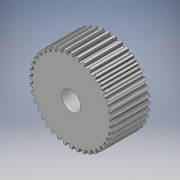
# Autodesk Inventor part: engranaje_grande_1
Saved by Autodesk Inventor 2017 (Build 210142000, 142)
## iProperties
Created: 2016-10-04
Part Number: engranaje_grande_1
Material: Generic
Document SubType Name: Modeling
Designer: ANDRES
Density: 1 g/cm^3
Appearance: Default
Author: ANDRES
Autodesk Inventor part; units mm, degrees
(part 1 of 2)
ref_plane "YZ Plane" through (0, 0, 0) normal (1, 0, 0) x (0, 1, 0)
ref_plane "XZ Plane" through (0, 0, 0) normal (0, 1, 0) x (-1, 0, 0)
ref_plane "XY Plane" through (0, 0, 0) normal (0, 0, 1) x (1, 0, 0)
sketch "Sketch1" plane through (0, 0, 0) normal (0, 1, 0) x (-1, 0, 0)
  line L0 (2.1221, 1.1536) -> (2.1255, 1.153)
  line L1 (2.1255, 1.153) -> (2.1288, 1.1523)
  line L2 (2.1288, 1.1523) -> (2.1356, 1.1509)
  line L3 (2.1356, 1.1509) -> (2.1491, 1.1475)
  line L4 (2.1491, 1.1475) -> (2.1626, 1.1435)
  line L5 (2.1626, 1.1435) -> (2.1761, 1.1388)
  line L6 (2.1761, 1.1388) -> (2.1896, 1.1337)
  line L7 (2.1896, 1.1337) -> (2.2031, 1.128)
  line L8 (2.2031, 1.128) -> (2.2031, 1.0754)
  line L9 (2.2031, 1.0754) -> (2.1896, 1.0697)
  line L10 (2.1896, 1.0697) -> (2.1761, 1.0646)
  line L11 (2.1761, 1.0646) -> (2.1626, 1.06)
  line L12 (2.1626, 1.06) -> (2.1491, 1.0559)
  line L13 (2.1491, 1.0559) -> (2.1356, 1.0525)
  line L14 (2.1356, 1.0525) -> (2.1288, 1.0511)
  line L15 (2.1288, 1.0511) -> (2.1255, 1.0505)
  line L16 (2.1255, 1.0505) -> (2.1221, 1.0499)
  line L17 (2.1221, 1.0499) -> (2.1176, 0.9933)
  line L18 (2.1176, 0.9933) -> (2.1209, 0.9922)
  line L19 (2.1209, 0.9922) -> (2.1241, 0.991)
  line L20 (2.1241, 0.991) -> (2.1305, 0.9885)
  line L21 (2.1305, 0.9885) -> (2.1433, 0.9831)
  line L22 (2.1433, 0.9831) -> (2.1561, 0.977)
  line L23 (2.1561, 0.977) -> (2.1687, 0.9703)
  line L24 (2.1687, 0.9703) -> (2.1812, 0.9631)
  line L25 (2.1812, 0.9631) -> (2.1936, 0.9554)
  line L26 (2.1936, 0.9554) -> (2.1854, 0.9034)
  line L27 (2.1854, 0.9034) -> (2.1712, 0.8999)
  line L28 (2.1712, 0.8999) -> (2.1571, 0.897)
  line L29 (2.1571, 0.897) -> (2.143, 0.8945)
  line L30 (2.143, 0.8945) -> (2.129, 0.8926)
  line L31 (2.129, 0.8926) -> (2.1151, 0.8914)
  line L32 (2.1151, 0.8914) -> (2.1083, 0.891)
  line L33 (2.1083, 0.891) -> (2.1048, 0.8909)
  line L34 (2.1048, 0.8909) -> (2.1014, 0.8909)
  line L35 (2.1014, 0.8909) -> (2.0882, 0.8357)
  line L36 (2.0882, 0.8357) -> (2.0912, 0.8341)
  line L37 (2.0912, 0.8341) -> (2.0942, 0.8324)
  line L38 (2.0942, 0.8324) -> (2.1002, 0.829)
  line L39 (2.1002, 0.829) -> (2.112, 0.8216)
  line L40 (2.112, 0.8216) -> (2.1236, 0.8136)
  line L41 (2.1236, 0.8136) -> (2.135, 0.805)
  line L42 (2.135, 0.805) -> (2.1462, 0.7959)
  line L43 (2.1462, 0.7959) -> (2.1573, 0.7864)
  line L44 (2.1573, 0.7864) -> (2.1411, 0.7363)
  line L45 (2.1411, 0.7363) -> (2.1265, 0.7351)
  line L46 (2.1265, 0.7351) -> (2.112, 0.7344)
  line L47 (2.112, 0.7344) -> (2.0978, 0.7342)
  line L48 (2.0978, 0.7342) -> (2.0837, 0.7345)
  line L49 (2.0837, 0.7345) -> (2.0698, 0.7355)
  line L50 (2.0698, 0.7355) -> (2.0629, 0.7362)
  line L51 (2.0629, 0.7362) -> (2.0595, 0.7366)
  line L52 (2.0595, 0.7366) -> (2.0561, 0.7371)
  line L53 (2.0561, 0.7371) -> (2.0344, 0.6847)
  line L54 (2.0344, 0.6847) -> (2.0371, 0.6826)
  line L55 (2.0371, 0.6826) -> (2.0398, 0.6805)
  line L56 (2.0398, 0.6805) -> (2.0452, 0.6762)
  line L57 (2.0452, 0.6762) -> (2.0557, 0.667)
  line L58 (2.0557, 0.667) -> (2.0659, 0.6573)
  line L59 (2.0659, 0.6573) -> (2.0759, 0.647)
  line L60 (2.0759, 0.647) -> (2.0856, 0.6363)
  line L61 (2.0856, 0.6363) -> (2.095, 0.6251)
  line L62 (2.095, 0.6251) -> (2.0711, 0.5783)
  line L63 (2.0711, 0.5783) -> (2.0565, 0.5793)
  line L64 (2.0565, 0.5793) -> (2.0421, 0.5808)
  line L65 (2.0421, 0.5808) -> (2.028, 0.5829)
  line L66 (2.028, 0.5829) -> (2.0141, 0.5854)
  line L67 (2.0141, 0.5854) -> (2.0006, 0.5885)
  line L68 (2.0006, 0.5885) -> (1.9939, 0.5903)
  line L69 (1.9939, 0.5903) -> (1.9906, 0.5913)
  line L70 (1.9906, 0.5913) -> (1.9873, 0.5923)
  line L71 (1.9873, 0.5923) -> (1.9577, 0.5439)
  line L72 (1.9577, 0.5439) -> (1.9601, 0.5414)
  line L73 (1.9601, 0.5414) -> (1.9624, 0.5389)
  line L74 (1.9624, 0.5389) -> (1.967, 0.5338)
  line L75 (1.967, 0.5338) -> (1.976, 0.5231)
  line L76 (1.976, 0.5231) -> (1.9845, 0.5119)
  line L77 (1.9845, 0.5119) -> (1.9927, 0.5002)
  line L78 (1.9927, 0.5002) -> (2.0006, 0.4881)
  line L79 (2.0006, 0.4881) -> (2.0082, 0.4756)
  line L80 (2.0082, 0.4756) -> (1.9773, 0.4331)
  line L81 (1.9773, 0.4331) -> (1.963, 0.4364)
  line L82 (1.963, 0.4364) -> (1.9491, 0.4401)
  line L83 (1.9491, 0.4401) -> (1.9354, 0.4444)
  line L84 (1.9354, 0.4444) -> (1.9221, 0.449)
  line L85 (1.9221, 0.449) -> (1.9092, 0.4542)
  line L86 (1.9092, 0.4542) -> (1.9029, 0.457)
  line L87 (1.9029, 0.457) -> (1.8998, 0.4585)
  line L88 (1.8998, 0.4585) -> (1.8967, 0.46)
  line L89 (1.8967, 0.46) -> (1.8599, 0.4168)
  line L90 (1.8599, 0.4168) -> (1.8619, 0.414)
  line L91 (1.8619, 0.414) -> (1.8638, 0.4112)
  line L92 (1.8638, 0.4112) -> (1.8675, 0.4054)
  line L93 (1.8675, 0.4054) -> (1.8747, 0.3935)
  line L94 (1.8747, 0.3935) -> (1.8814, 0.3811)
  line L95 (1.8814, 0.3811) -> (1.8877, 0.3683)
  line L96 (1.8877, 0.3683) -> (1.8936, 0.3551)
  line L97 (1.8936, 0.3551) -> (1.8991, 0.3415)
  line L98 (1.8991, 0.3415) -> (1.8619, 0.3043)
  line L99 (1.8619, 0.3043) -> (1.8484, 0.3098)
  line L100 (1.8484, 0.3098) -> (1.8352, 0.3157)
  line L101 (1.8352, 0.3157) -> (1.8223, 0.322)
  line L102 (1.8223, 0.322) -> (1.8099, 0.3287)
  line L103 (1.8099, 0.3287) -> (1.798, 0.3359)
  line L104 (1.798, 0.3359) -> (1.7922, 0.3396)
  line L105 (1.7922, 0.3396) -> (1.7894, 0.3416)
  line L106 (1.7894, 0.3416) -> (1.7866, 0.3435)
  line L107 (1.7866, 0.3435) -> (1.7434, 0.3067)
  line L108 (1.7434, 0.3067) -> (1.7449, 0.3036)
  line L109 (1.7449, 0.3036) -> (1.7464, 0.3005)
  line L110 (1.7464, 0.3005) -> (1.7492, 0.2942)
  line L111 (1.7492, 0.2942) -> (1.7544, 0.2813)
  line L112 (1.7544, 0.2813) -> (1.7591, 0.268)
  line L113 (1.7591, 0.268) -> (1.7633, 0.2543)
  line L114 (1.7633, 0.2543) -> (1.767, 0.2404)
  line L115 (1.767, 0.2404) -> (1.7704, 0.2261)
  line L116 (1.7704, 0.2261) -> (1.7278, 0.1952)
  line L117 (1.7278, 0.1952) -> (1.7153, 0.2028)
  line L118 (1.7153, 0.2028) -> (1.7032, 0.2107)
  line L119 (1.7032, 0.2107) -> (1.6915, 0.2189)
  line L120 (1.6915, 0.2189) -> (1.6803, 0.2275)
  line L121 (1.6803, 0.2275) -> (1.6696, 0.2364)
  line L122 (1.6696, 0.2364) -> (1.6645, 0.241)
  line L123 (1.6645, 0.241) -> (1.662, 0.2434)
  line L124 (1.662, 0.2434) -> (1.6595, 0.2457)
  line L125 (1.6595, 0.2457) -> (1.6112, 0.2161)
  line L126 (1.6112, 0.2161) -> (1.6121, 0.2128)
  line L127 (1.6121, 0.2128) -> (1.6131, 0.2095)
  line L128 (1.6131, 0.2095) -> (1.6149, 0.2029)
  line L129 (1.6149, 0.2029) -> (1.618, 0.1893)
  line L130 (1.618, 0.1893) -> (1.6205, 0.1754)
  line L131 (1.6205, 0.1754) -> (1.6226, 0.1613)
  line L132 (1.6226, 0.1613) -> (1.6241, 0.1469)
  line L133 (1.6241, 0.1469) -> (1.6252, 0.1323)
  line L134 (1.6252, 0.1323) -> (1.5783, 0.1084)
  line L135 (1.5783, 0.1084) -> (1.5671, 0.1179)
  line L136 (1.5671, 0.1179) -> (1.5564, 0.1275)
  line L137 (1.5564, 0.1275) -> (1.5461, 0.1375)
  line L138 (1.5461, 0.1375) -> (1.5364, 0.1477)
  line L139 (1.5364, 0.1477) -> (1.5273, 0.1582)
  line L140 (1.5273, 0.1582) -> (1.5229, 0.1636)
  line L141 (1.5229, 0.1636) -> (1.5208, 0.1663)
  line L142 (1.5208, 0.1663) -> (1.5188, 0.169)
  line L143 (1.5188, 0.169) -> (1.4663, 0.1473)
  line L144 (1.4663, 0.1473) -> (1.4668, 0.1439)
  line L145 (1.4668, 0.1439) -> (1.4672, 0.1405)
  line L146 (1.4672, 0.1405) -> (1.468, 0.1336)
  line L147 (1.468, 0.1336) -> (1.4689, 0.1197)
  line L148 (1.4689, 0.1197) -> (1.4692, 0.1056)
  line L149 (1.4692, 0.1056) -> (1.469, 0.0914)
  line L150 (1.469, 0.0914) -> (1.4683, 0.0769)
  line L151 (1.4683, 0.0769) -> (1.4671, 0.0624)
  line L152 (1.4671, 0.0624) -> (1.417, 0.0461)
  line L153 (1.417, 0.0461) -> (1.4075, 0.0572)
  line L154 (1.4075, 0.0572) -> (1.3984, 0.0684)
  line L155 (1.3984, 0.0684) -> (1.3898, 0.0799)
  line L156 (1.3898, 0.0799) -> (1.3818, 0.0915)
  line L157 (1.3818, 0.0915) -> (1.3744, 0.1033)
  line L158 (1.3744, 0.1033) -> (1.371, 0.1092)
  line L159 (1.371, 0.1092) -> (1.3693, 0.1122)
  line L160 (1.3693, 0.1122) -> (1.3677, 0.1153)
  line L161 (1.3677, 0.1153) -> (1.3125, 0.102)
  line L162 (1.3125, 0.102) -> (1.3125, 0.0986)
  line L163 (1.3125, 0.0986) -> (1.3124, 0.0952)
  line L164 (1.3124, 0.0952) -> (1.312, 0.0883)
  line L165 (1.312, 0.0883) -> (1.3108, 0.0744)
  line L166 (1.3108, 0.0744) -> (1.3089, 0.0604)
  line L167 (1.3089, 0.0604) -> (1.3065, 0.0464)
  line L168 (1.3065, 0.0464) -> (1.3035, 0.0322)
  line L169 (1.3035, 0.0322) -> (1.3, 0.018)
  line L170 (1.3, 0.018) -> (1.248, 0.0098)
  line L171 (1.248, 0.0098) -> (1.2403, 0.0222)
  line L172 (1.2403, 0.0222) -> (1.2331, 0.0347)
  line L173 (1.2331, 0.0347) -> (1.2264, 0.0474)
  line L174 (1.2264, 0.0474) -> (1.2203, 0.0601)
  line L175 (1.2203, 0.0601) -> (1.2149, 0.0729)
  line L176 (1.2149, 0.0729) -> (1.2124, 0.0793)
  line L177 (1.2124, 0.0793) -> (1.2112, 0.0825)
  line L178 (1.2112, 0.0825) -> (1.2101, 0.0858)
  line L179 (1.2101, 0.0858) -> (1.1536, 0.0813)
  line L180 (1.1536, 0.0813) -> (1.153, 0.078)
  line L181 (1.153, 0.078) -> (1.1523, 0.0746)
  line L182 (1.1523, 0.0746) -> (1.1509, 0.0678)
  line L183 (1.1509, 0.0678) -> (1.1475, 0.0543)
  line L184 (1.1475, 0.0543) -> (1.1435, 0.0408)
  line L185 (1.1435, 0.0408) -> (1.1388, 0.0273)
  line L186 (1.1388, 0.0273) -> (1.1337, 0.0138)
  line L187 (1.1337, 0.0138) -> (1.128, 0.0003)
  line L188 (1.128, 0.0003) -> (1.0754, 0.0003)
  line L189 (1.0754, 0.0003) -> (1.0697, 0.0138)
  line L190 (1.0697, 0.0138) -> (1.0646, 0.0273)
  line L191 (1.0646, 0.0273) -> (1.06, 0.0408)
  line L192 (1.06, 0.0408) -> (1.0559, 0.0543)
  line L193 (1.0559, 0.0543) -> (1.0525, 0.0678)
  line L194 (1.0525, 0.0678) -> (1.0511, 0.0746)
  line L195 (1.0511, 0.0746) -> (1.0505, 0.078)
  line L196 (1.0505, 0.078) -> (1.0499, 0.0813)
  line L197 (1.0499, 0.0813) -> (0.9933, 0.0858)
  line L198 (0.9933, 0.0858) -> (0.9922, 0.0825)
  line L199 (0.9922, 0.0825) -> (0.991, 0.0793)
  line L200 (0.991, 0.0793) -> (0.9885, 0.0729)
  line L201 (0.9885, 0.0729) -> (0.9831, 0.0601)
  line L202 (0.9831, 0.0601) -> (0.977, 0.0474)
  line L203 (0.977, 0.0474) -> (0.9703, 0.0347)
  line L204 (0.9703, 0.0347) -> (0.9631, 0.0222)
  line L205 (0.9631, 0.0222) -> (0.9554, 0.0098)
  line L206 (0.9554, 0.0098) -> (0.9034, 0.018)
  line L207 (0.9034, 0.018) -> (0.8999, 0.0322)
  line L208 (0.8999, 0.0322) -> (0.897, 0.0464)
  line L209 (0.897, 0.0464) -> (0.8945, 0.0604)
  line L210 (0.8945, 0.0604) -> (0.8926, 0.0744)
  line L211 (0.8926, 0.0744) -> (0.8914, 0.0883)
  line L212 (0.8914, 0.0883) -> (0.891, 0.0952)
  line L213 (0.891, 0.0952) -> (0.8909, 0.0986)
  line L214 (0.8909, 0.0986) -> (0.8909, 0.102)
  line L215 (0.8909, 0.102) -> (0.8357, 0.1153)
  line L216 (0.8357, 0.1153) -> (0.8341, 0.1122)
  line L217 (0.8341, 0.1122) -> (0.8324, 0.1092)
  line L218 (0.8324, 0.1092) -> (0.829, 0.1033)
  line L219 (0.829, 0.1033) -> (0.8216, 0.0915)
  line L220 (0.8216, 0.0915) -> (0.8136, 0.0799)
  line L221 (0.8136, 0.0799) -> (0.805, 0.0684)
  line L222 (0.805, 0.0684) -> (0.7959, 0.0572)
  line L223 (0.7959, 0.0572) -> (0.7864, 0.0461)
  line L224 (0.7864, 0.0461) -> (0.7363, 0.0624)
  line L225 (0.7363, 0.0624) -> (0.7351, 0.0769)
  line L226 (0.7351, 0.0769) -> (0.7344, 0.0914)
  line L227 (0.7344, 0.0914) -> (0.7342, 0.1056)
  line L228 (0.7342, 0.1056) -> (0.7345, 0.1197)
  line L229 (0.7345, 0.1197) -> (0.7355, 0.1336)
  line L230 (0.7355, 0.1336) -> (0.7362, 0.1405)
  line L231 (0.7362, 0.1405) -> (0.7366, 0.1439)
  line L232 (0.7366, 0.1439) -> (0.7371, 0.1473)
  line L233 (0.7371, 0.1473) -> (0.6847, 0.169)
  line L234 (0.6847, 0.169) -> (0.6826, 0.1663)
  line L235 (0.6826, 0.1663) -> (0.6805, 0.1636)
  line L236 (0.6805, 0.1636) -> (0.6762, 0.1582)
  line L237 (0.6762, 0.1582) -> (0.667, 0.1477)
  line L238 (0.667, 0.1477) -> (0.6573, 0.1375)
  line L239 (0.6573, 0.1375) -> (0.647, 0.1275)
  line L240 (0.647, 0.1275) -> (0.6363, 0.1179)
  line L241 (0.6363, 0.1179) -> (0.6251, 0.1084)
  line L242 (0.6251, 0.1084) -> (0.5783, 0.1323)
  line L243 (0.5783, 0.1323) -> (0.5793, 0.1469)
  line L244 (0.5793, 0.1469) -> (0.5808, 0.1613)
  line L245 (0.5808, 0.1613) -> (0.5829, 0.1754)
  line L246 (0.5829, 0.1754) -> (0.5854, 0.1893)
  line L247 (0.5854, 0.1893) -> (0.5885, 0.2029)
  line L248 (0.5885, 0.2029) -> (0.5903, 0.2095)
  line L249 (0.5903, 0.2095) -> (0.5913, 0.2128)
  line L250 (0.5913, 0.2128) -> (0.5923, 0.2161)
  line L251 (0.5923, 0.2161) -> (0.5439, 0.2457)
  line L252 (0.5439, 0.2457) -> (0.5414, 0.2434)
  line L253 (0.5414, 0.2434) -> (0.5389, 0.241)
  line L254 (0.5389, 0.241) -> (0.5338, 0.2364)
  line L255 (0.5338, 0.2364) -> (0.5231, 0.2275)
  line L256 (0.5231, 0.2275) -> (0.5119, 0.2189)
  line L257 (0.5119, 0.2189) -> (0.5002, 0.2107)
  line L258 (0.5002, 0.2107) -> (0.4881, 0.2028)
  line L259 (0.4881, 0.2028) -> (0.4756, 0.1952)
  line L260 (0.4756, 0.1952) -> (0.4331, 0.2261)
  line L261 (0.4331, 0.2261) -> (0.4364, 0.2404)
  line L262 (0.4364, 0.2404) -> (0.4401, 0.2543)
  line L263 (0.4401, 0.2543) -> (0.4444, 0.268)
  line L264 (0.4444, 0.268) -> (0.449, 0.2813)
  line L265 (0.449, 0.2813) -> (0.4542, 0.2942)
  line L266 (0.4542, 0.2942) -> (0.457, 0.3005)
  line L267 (0.457, 0.3005) -> (0.4585, 0.3036)
  line L268 (0.4585, 0.3036) -> (0.46, 0.3067)
  line L269 (0.46, 0.3067) -> (0.4168, 0.3435)
  line L270 (0.4168, 0.3435) -> (0.414, 0.3416)
  line L271 (0.414, 0.3416) -> (0.4112, 0.3396)
  line L272 (0.4112, 0.3396) -> (0.4054, 0.3359)
  line L273 (0.4054, 0.3359) -> (0.3935, 0.3287)
  line L274 (0.3935, 0.3287) -> (0.3811, 0.322)
  line L275 (0.3811, 0.322) -> (0.3683, 0.3157)
  line L276 (0.3683, 0.3157) -> (0.3551, 0.3098)
  line L277 (0.3551, 0.3098) -> (0.3415, 0.3043)
  line L278 (0.3415, 0.3043) -> (0.3043, 0.3415)
  line L279 (0.3043, 0.3415) -> (0.3098, 0.3551)
  line L280 (0.3098, 0.3551) -> (0.3157, 0.3683)
  line L281 (0.3157, 0.3683) -> (0.322, 0.3811)
  line L282 (0.322, 0.3811) -> (0.3287, 0.3935)
  line L283 (0.3287, 0.3935) -> (0.3359, 0.4054)
  line L284 (0.3359, 0.4054) -> (0.3396, 0.4112)
  line L285 (0.3396, 0.4112) -> (0.3416, 0.414)
  line L286 (0.3416, 0.414) -> (0.3435, 0.4168)
  line L287 (0.3435, 0.4168) -> (0.3067, 0.46)
  line L288 (0.3067, 0.46) -> (0.3036, 0.4585)
  line L289 (0.3036, 0.4585) -> (0.3005, 0.457)
  line L290 (0.3005, 0.457) -> (0.2942, 0.4542)
  line L291 (0.2942, 0.4542) -> (0.2813, 0.449)
  line L292 (0.2813, 0.449) -> (0.268, 0.4444)
  line L293 (0.268, 0.4444) -> (0.2543, 0.4401)
  line L294 (0.2543, 0.4401) -> (0.2404, 0.4364)
  line L295 (0.2404, 0.4364) -> (0.2261, 0.4331)
  line L296 (0.2261, 0.4331) -> (0.1952, 0.4756)
  line L297 (0.1952, 0.4756) -> (0.2028, 0.4881)
  line L298 (0.2028, 0.4881) -> (0.2107, 0.5002)
  line L299 (0.2107, 0.5002) -> (0.2189, 0.5119)
  line L300 (0.2189, 0.5119) -> (0.2275, 0.5231)
  line L301 (0.2275, 0.5231) -> (0.2364, 0.5338)
  line L302 (0.2364, 0.5338) -> (0.241, 0.5389)
  line L303 (0.241, 0.5389) -> (0.2434, 0.5414)
  line L304 (0.2434, 0.5414) -> (0.2457, 0.5439)
  line L305 (0.2457, 0.5439) -> (0.2161, 0.5923)
  line L306 (0.2161, 0.5923) -> (0.2128, 0.5913)
  line L307 (0.2128, 0.5913) -> (0.2095, 0.5903)
  line L308 (0.2095, 0.5903) -> (0.2029, 0.5885)
  line L309 (0.2029, 0.5885) -> (0.1893, 0.5854)
  line L310 (0.1893, 0.5854) -> (0.1754, 0.5829)
  line L311 (0.1754, 0.5829) -> (0.1613, 0.5808)
  line L312 (0.1613, 0.5808) -> (0.1469, 0.5793)
  line L313 (0.1469, 0.5793) -> (0.1323, 0.5783)
  line L314 (0.1323, 0.5783) -> (0.1084, 0.6251)
  line L315 (0.1084, 0.6251) -> (0.1179, 0.6363)
  line L316 (0.1179, 0.6363) -> (0.1275, 0.647)
  line L317 (0.1275, 0.647) -> (0.1375, 0.6573)
  line L318 (0.1375, 0.6573) -> (0.1477, 0.667)
  line L319 (0.1477, 0.667) -> (0.1582, 0.6762)
  line L320 (0.1582, 0.6762) -> (0.1636, 0.6805)
  line L321 (0.1636, 0.6805) -> (0.1663, 0.6826)
  line L322 (0.1663, 0.6826) -> (0.169, 0.6847)
  line L323 (0.169, 0.6847) -> (0.1473, 0.7371)
  line L324 (0.1473, 0.7371) -> (0.1439, 0.7366)
  line L325 (0.1439, 0.7366) -> (0.1405, 0.7362)
  line L326 (0.1405, 0.7362) -> (0.1336, 0.7355)
  line L327 (0.1336, 0.7355) -> (0.1197, 0.7345)
  line L328 (0.1197, 0.7345) -> (0.1056, 0.7342)
  line L329 (0.1056, 0.7342) -> (0.0914, 0.7344)
  line L330 (0.0914, 0.7344) -> (0.0769, 0.7351)
  line L331 (0.0769, 0.7351) -> (0.0624, 0.7363)
  line L332 (0.0624, 0.7363) -> (0.0461, 0.7864)
  line L333 (0.0461, 0.7864) -> (0.0572, 0.7959)
  line L334 (0.0572, 0.7959) -> (0.0684, 0.805)
  line L335 (0.0684, 0.805) -> (0.0799, 0.8136)
  line L336 (0.0799, 0.8136) -> (0.0915, 0.8216)
  line L337 (0.0915, 0.8216) -> (0.1033, 0.829)
  line L338 (0.1033, 0.829) -> (0.1092, 0.8324)
  line L339 (0.1092, 0.8324) -> (0.1122, 0.8341)
  line L340 (0.1122, 0.8341) -> (0.1153, 0.8357)
  line L341 (0.1153, 0.8357) -> (0.102, 0.8909)
  line L342 (0.102, 0.8909) -> (0.0986, 0.8909)
  line L343 (0.0986, 0.8909) -> (0.0952, 0.891)
  line L344 (0.0952, 0.891) -> (0.0883, 0.8914)
  line L345 (0.0883, 0.8914) -> (0.0744, 0.8926)
  line L346 (0.0744, 0.8926) -> (0.0604, 0.8945)
  line L347 (0.0604, 0.8945) -> (0.0464, 0.897)
  line L348 (0.0464, 0.897) -> (0.0322, 0.8999)
  line L349 (0.0322, 0.8999) -> (0.018, 0.9034)
  line L350 (0.018, 0.9034) -> (0.0098, 0.9554)
  line L351 (0.0098, 0.9554) -> (0.0222, 0.9631)
  line L352 (0.0222, 0.9631) -> (0.0347, 0.9703)
  line L353 (0.0347, 0.9703) -> (0.0474, 0.977)
  line L354 (0.0474, 0.977) -> (0.0601, 0.9831)
  line L355 (0.0601, 0.9831) -> (0.0729, 0.9885)
  line L356 (0.0729, 0.9885) -> (0.0793, 0.991)
  line L357 (0.0793, 0.991) -> (0.0825, 0.9922)
  line L358 (0.0825, 0.9922) -> (0.0858, 0.9933)
  line L359 (0.0858, 0.9933) -> (0.0813, 1.0499)
  line L360 (0.0813, 1.0499) -> (0.078, 1.0505)
  line L361 (0.078, 1.0505) -> (0.0746, 1.0511)
  line L362 (0.0746, 1.0511) -> (0.0678, 1.0525)
  line L363 (0.0678, 1.0525) -> (0.0543, 1.0559)
  line L364 (0.0543, 1.0559) -> (0.0408, 1.06)
  line L365 (0.0408, 1.06) -> (0.0273, 1.0646)
  line L366 (0.0273, 1.0646) -> (0.0138, 1.0697)
  line L367 (0.0138, 1.0697) -> (0.0003, 1.0754)
  line L368 (0.0003, 1.0754) -> (0.0003, 1.128)
  line L369 (0.0003, 1.128) -> (0.0138, 1.1337)
  line L370 (0.0138, 1.1337) -> (0.0273, 1.1388)
  line L371 (0.0273, 1.1388) -> (0.0408, 1.1435)
  line L372 (0.0408, 1.1435) -> (0.0543, 1.1475)
  line L373 (0.0543, 1.1475) -> (0.0678, 1.1509)
  line L374 (0.0678, 1.1509) -> (0.0746, 1.1523)
  line L375 (0.0746, 1.1523) -> (0.078, 1.153)
  line L376 (0.078, 1.153) -> (0.0813, 1.1536)
  line L377 (0.0813, 1.1536) -> (0.0858, 1.2101)
  line L378 (0.0858, 1.2101) -> (0.0825, 1.2112)
  line L379 (0.0825, 1.2112) -> (0.0793, 1.2124)
  line L380 (0.0793, 1.2124) -> (0.0729, 1.2149)
  line L381 (0.0729, 1.2149) -> (0.0601, 1.2203)
  line L382 (0.0601, 1.2203) -> (0.0474, 1.2264)
  line L383 (0.0474, 1.2264) -> (0.0347, 1.2331)
  line L384 (0.0347, 1.2331) -> (0.0222, 1.2403)
  line L385 (0.0222, 1.2403) -> (0.0098, 1.248)
  line L386 (0.0098, 1.248) -> (0.018, 1.3)
  line L387 (0.018, 1.3) -> (0.0322, 1.3035)
  line L388 (0.0322, 1.3035) -> (0.0464, 1.3065)
  line L389 (0.0464, 1.3065) -> (0.0604, 1.3089)
  line L390 (0.0604, 1.3089) -> (0.0744, 1.3108)
  line L391 (0.0744, 1.3108) -> (0.0883, 1.312)
  line L392 (0.0883, 1.312) -> (0.0952, 1.3124)
  line L393 (0.0952, 1.3124) -> (0.0986, 1.3125)
  line L394 (0.0986, 1.3125) -> (0.102, 1.3125)
  line L395 (0.102, 1.3125) -> (0.1153, 1.3677)
  line L396 (0.1153, 1.3677) -> (0.1122, 1.3693)
  line L397 (0.1122, 1.3693) -> (0.1092, 1.371)
  line L398 (0.1092, 1.371) -> (0.1033, 1.3744)
  line L399 (0.1033, 1.3744) -> (0.0915, 1.3818)
  line L400 (0.0915, 1.3818) -> (0.0799, 1.3898)
  line L401 (0.0799, 1.3898) -> (0.0684, 1.3984)
  line L402 (0.0684, 1.3984) -> (0.0572, 1.4075)
  line L403 (0.0572, 1.4075) -> (0.0461, 1.417)
  line L404 (0.0461, 1.417) -> (0.0624, 1.4671)
  line L405 (0.0624, 1.4671) -> (0.0769, 1.4683)
  line L406 (0.0769, 1.4683) -> (0.0914, 1.469)
  line L407 (0.0914, 1.469) -> (0.1056, 1.4692)
  line L408 (0.1056, 1.4692) -> (0.1197, 1.4689)
  line L409 (0.1197, 1.4689) -> (0.1336, 1.468)
  line L410 (0.1336, 1.468) -> (0.1405, 1.4672)
  line L411 (0.1405, 1.4672) -> (0.1439, 1.4668)
  line L412 (0.1439, 1.4668) -> (0.1473, 1.4663)
  line L413 (0.1473, 1.4663) -> (0.169, 1.5188)
  line L414 (0.169, 1.5188) -> (0.1663, 1.5208)
  line L415 (0.1663, 1.5208) -> (0.1636, 1.5229)
  line L416 (0.1636, 1.5229) -> (0.1582, 1.5273)
  line L417 (0.1582, 1.5273) -> (0.1477, 1.5364)
  line L418 (0.1477, 1.5364) -> (0.1375, 1.5461)
  line L419 (0.1375, 1.5461) -> (0.1275, 1.5564)
  line L420 (0.1275, 1.5564) -> (0.1179, 1.5671)
  line L421 (0.1179, 1.5671) -> (0.1084, 1.5783)
  line L422 (0.1084, 1.5783) -> (0.1323, 1.6252)
  line L423 (0.1323, 1.6252) -> (0.1469, 1.6241)
  line L424 (0.1469, 1.6241) -> (0.1613, 1.6226)
  line L425 (0.1613, 1.6226) -> (0.1754, 1.6205)
  line L426 (0.1754, 1.6205) -> (0.1893, 1.618)
  line L427 (0.1893, 1.618) -> (0.2029, 1.6149)
  line L428 (0.2029, 1.6149) -> (0.2095, 1.6131)
  line L429 (0.2095, 1.6131) -> (0.2128, 1.6121)
  line L430 (0.2128, 1.6121) -> (0.2161, 1.6112)
  line L431 (0.2161, 1.6112) -> (0.2457, 1.6595)
  line L432 (0.2457, 1.6595) -> (0.2434, 1.662)
  line L433 (0.2434, 1.662) -> (0.241, 1.6645)
  line L434 (0.241, 1.6645) -> (0.2364, 1.6696)
  line L435 (0.2364, 1.6696) -> (0.2275, 1.6803)
  line L436 (0.2275, 1.6803) -> (0.2189, 1.6915)
  line L437 (0.2189, 1.6915) -> (0.2107, 1.7032)
  line L438 (0.2107, 1.7032) -> (0.2028, 1.7153)
  line L439 (0.2028, 1.7153) -> (0.1952, 1.7278)
  line L440 (0.1952, 1.7278) -> (0.2261, 1.7704)
  line L441 (0.2261, 1.7704) -> (0.2404, 1.767)
  line L442 (0.2404, 1.767) -> (0.2543, 1.7633)
  line L443 (0.2543, 1.7633) -> (0.268, 1.7591)
  line L444 (0.268, 1.7591) -> (0.2813, 1.7544)
  line L445 (0.2813, 1.7544) -> (0.2942, 1.7492)
  line L446 (0.2942, 1.7492) -> (0.3005, 1.7464)
  line L447 (0.3005, 1.7464) -> (0.3036, 1.7449)
  line L448 (0.3036, 1.7449) -> (0.3067, 1.7434)
  line L449 (0.3067, 1.7434) -> (0.3435, 1.7866)
  line L450 (0.3435, 1.7866) -> (0.3416, 1.7894)
  line L451 (0.3416, 1.7894) -> (0.3396, 1.7922)
  line L452 (0.3396, 1.7922) -> (0.3359, 1.798)
  line L453 (0.3359, 1.798) -> (0.3287, 1.8099)
  line L454 (0.3287, 1.8099) -> (0.322, 1.8223)
  line L455 (0.322, 1.8223) -> (0.3157, 1.8352)
  line L456 (0.3157, 1.8352) -> (0.3098, 1.8484)
  line L457 (0.3098, 1.8484) -> (0.3043, 1.8619)
  line L458 (0.3043, 1.8619) -> (0.3415, 1.8991)
  line L459 (0.3415, 1.8991) -> (0.3551, 1.8936)
  line L460 (0.3551, 1.8936) -> (0.3683, 1.8877)
  line L461 (0.3683, 1.8877) -> (0.3811, 1.8814)
  line L462 (0.3811, 1.8814) -> (0.3935, 1.8747)
  line L463 (0.3935, 1.8747) -> (0.4054, 1.8675)
  line L464 (0.4054, 1.8675) -> (0.4112, 1.8638)
  line L465 (0.4112, 1.8638) -> (0.414, 1.8619)
  line L466 (0.414, 1.8619) -> (0.4168, 1.8599)
  line L467 (0.4168, 1.8599) -> (0.46, 1.8967)
  line L468 (0.46, 1.8967) -> (0.4585, 1.8998)
  line L469 (0.4585, 1.8998) -> (0.457, 1.9029)
  line L470 (0.457, 1.9029) -> (0.4542, 1.9092)
  line L471 (0.4542, 1.9092) -> (0.449, 1.9221)
  line L472 (0.449, 1.9221) -> (0.4444, 1.9354)
  line L473 (0.4444, 1.9354) -> (0.4401, 1.9491)
  line L474 (0.4401, 1.9491) -> (0.4364, 1.963)
  line L475 (0.4364, 1.963) -> (0.4331, 1.9773)
  line L476 (0.4331, 1.9773) -> (0.4756, 2.0082)
  line L477 (0.4756, 2.0082) -> (0.4881, 2.0006)
  line L478 (0.4881, 2.0006) -> (0.5002, 1.9927)
  line L479 (0.5002, 1.9927) -> (0.5119, 1.9845)
  line L480 (0.5119, 1.9845) -> (0.5231, 1.976)
  line L481 (0.5231, 1.976) -> (0.5338, 1.967)
  line L482 (0.5338, 1.967) -> (0.5389, 1.9624)
  line L483 (0.5389, 1.9624) -> (0.5414, 1.9601)
  line L484 (0.5414, 1.9601) -> (0.5439, 1.9577)
  line L485 (0.5439, 1.9577) -> (0.5923, 1.9873)
  line L486 (0.5923, 1.9873) -> (0.5913, 1.9906)
  line L487 (0.5913, 1.9906) -> (0.5903, 1.9939)
  line L488 (0.5903, 1.9939) -> (0.5885, 2.0006)
  line L489 (0.5885, 2.0006) -> (0.5854, 2.0141)
  line L490 (0.5854, 2.0141) -> (0.5829, 2.028)
  line L491 (0.5829, 2.028) -> (0.5808, 2.0421)
  line L492 (0.5808, 2.0421) -> (0.5793, 2.0565)
  line L493 (0.5793, 2.0565) -> (0.5783, 2.0711)
  line L494 (0.5783, 2.0711) -> (0.6251, 2.095)
  line L495 (0.6251, 2.095) -> (0.6363, 2.0856)
  line L496 (0.6363, 2.0856) -> (0.647, 2.0759)
  line L497 (0.647, 2.0759) -> (0.6573, 2.0659)
  line L498 (0.6573, 2.0659) -> (0.667, 2.0557)
  line L499 (0.667, 2.0557) -> (0.6762, 2.0452)
  line L500 (0.6762, 2.0452) -> (0.6805, 2.0398)
  line L501 (0.6805, 2.0398) -> (0.6826, 2.0371)
  line L502 (0.6826, 2.0371) -> (0.6847, 2.0344)
  line L503 (0.6847, 2.0344) -> (0.7371, 2.0561)
  line L504 (0.7371, 2.0561) -> (0.7366, 2.0595)
  line L505 (0.7366, 2.0595) -> (0.7362, 2.0629)
  line L506 (0.7362, 2.0629) -> (0.7355, 2.0698)
  line L507 (0.7355, 2.0698) -> (0.7345, 2.0837)
  line L508 (0.7345, 2.0837) -> (0.7342, 2.0978)
  line L509 (0.7342, 2.0978) -> (0.7344, 2.112)
  line L510 (0.7344, 2.112) -> (0.7351, 2.1265)
  line L511 (0.7351, 2.1265) -> (0.7363, 2.1411)
  line L512 (0.7363, 2.1411) -> (0.7864, 2.1573)
  line L513 (0.7864, 2.1573) -> (0.7959, 2.1462)
  line L514 (0.7959, 2.1462) -> (0.805, 2.135)
  line L515 (0.805, 2.135) -> (0.8136, 2.1236)
  line L516 (0.8136, 2.1236) -> (0.8216, 2.112)
  line L517 (0.8216, 2.112) -> (0.829, 2.1002)
  line L518 (0.829, 2.1002) -> (0.8324, 2.0942)
  line L519 (0.8324, 2.0942) -> (0.8341, 2.0912)
  line L520 (0.8341, 2.0912) -> (0.8357, 2.0882)
  line L521 (0.8357, 2.0882) -> (0.8909, 2.1014)
  line L522 (0.8909, 2.1014) -> (0.8909, 2.1048)
  line L523 (0.8909, 2.1048) -> (0.891, 2.1083)
  line L524 (0.891, 2.1083) -> (0.8914, 2.1151)
  line L525 (0.8914, 2.1151) -> (0.8926, 2.129)
  line L526 (0.8926, 2.129) -> (0.8945, 2.143)
  line L527 (0.8945, 2.143) -> (0.897, 2.1571)
  line L528 (0.897, 2.1571) -> (0.8999, 2.1712)
  line L529 (0.8999, 2.1712) -> (0.9034, 2.1854)
  line L530 (0.9034, 2.1854) -> (0.9554, 2.1936)
  line L531 (0.9554, 2.1936) -> (0.9631, 2.1812)
  line L532 (0.9631, 2.1812) -> (0.9703, 2.1687)
  line L533 (0.9703, 2.1687) -> (0.977, 2.1561)
  line L534 (0.977, 2.1561) -> (0.9831, 2.1433)
  line L535 (0.9831, 2.1433) -> (0.9885, 2.1305)
  line L536 (0.9885, 2.1305) -> (0.991, 2.1241)
  line L537 (0.991, 2.1241) -> (0.9922, 2.1209)
  line L538 (0.9922, 2.1209) -> (0.9933, 2.1176)
  line L539 (0.9933, 2.1176) -> (1.0499, 2.1221)
  line L540 (1.0499, 2.1221) -> (1.0505, 2.1255)
  line L541 (1.0505, 2.1255) -> (1.0511, 2.1288)
  line L542 (1.0511, 2.1288) -> (1.0525, 2.1356)
  line L543 (1.0525, 2.1356) -> (1.0559, 2.1491)
  line L544 (1.0559, 2.1491) -> (1.06, 2.1626)
  line L545 (1.06, 2.1626) -> (1.0646, 2.1761)
  line L546 (1.0646, 2.1761) -> (1.0697, 2.1896)
  line L547 (1.0697, 2.1896) -> (1.0754, 2.2031)
  line L548 (1.0754, 2.2031) -> (1.128, 2.2031)
  line L549 (1.128, 2.2031) -> (1.1337, 2.1896)
  line L550 (1.1337, 2.1896) -> (1.1388, 2.1761)
  line L551 (1.1388, 2.1761) -> (1.1435, 2.1626)
  line L552 (1.1435, 2.1626) -> (1.1475, 2.1491)
  line L553 (1.1475, 2.1491) -> (1.1509, 2.1356)
  line L554 (1.1509, 2.1356) -> (1.1523, 2.1288)
  line L555 (1.1523, 2.1288) -> (1.153, 2.1255)
  line L556 (1.153, 2.1255) -> (1.1536, 2.1221)
  line L557 (1.1536, 2.1221) -> (1.2101, 2.1176)
  line L558 (1.2101, 2.1176) -> (1.2112, 2.1209)
  line L559 (1.2112, 2.1209) -> (1.2124, 2.1241)
  line L560 (1.2124, 2.1241) -> (1.2149, 2.1305)
  line L561 (1.2149, 2.1305) -> (1.2203, 2.1433)
  line L562 (1.2203, 2.1433) -> (1.2264, 2.1561)
  line L563 (1.2264, 2.1561) -> (1.2331, 2.1687)
  line L564 (1.2331, 2.1687) -> (1.2403, 2.1812)
  line L565 (1.2403, 2.1812) -> (1.248, 2.1936)
  line L566 (1.248, 2.1936) -> (1.3, 2.1854)
  line L567 (1.3, 2.1854) -> (1.3035, 2.1712)
  line L568 (1.3035, 2.1712) -> (1.3065, 2.1571)
  line L569 (1.3065, 2.1571) -> (1.3089, 2.143)
  line L570 (1.3089, 2.143) -> (1.3108, 2.129)
  line L571 (1.3108, 2.129) -> (1.312, 2.1151)
  line L572 (1.312, 2.1151) -> (1.3124, 2.1083)
  line L573 (1.3124, 2.1083) -> (1.3125, 2.1048)
  line L574 (1.3125, 2.1048) -> (1.3125, 2.1014)
  line L575 (1.3125, 2.1014) -> (1.3677, 2.0882)
  line L576 (1.3677, 2.0882) -> (1.3693, 2.0912)
  line L577 (1.3693, 2.0912) -> (1.371, 2.0942)
  line L578 (1.371, 2.0942) -> (1.3744, 2.1002)
  line L579 (1.3744, 2.1002) -> (1.3818, 2.112)
  line L580 (1.3818, 2.112) -> (1.3898, 2.1236)
  line L581 (1.3898, 2.1236) -> (1.3984, 2.135)
  line L582 (1.3984, 2.135) -> (1.4075, 2.1462)
  line L583 (1.4075, 2.1462) -> (1.417, 2.1573)
  line L584 (1.417, 2.1573) -> (1.4671, 2.1411)
  line L585 (1.4671, 2.1411) -> (1.4683, 2.1265)
  line L586 (1.4683, 2.1265) -> (1.469, 2.112)
  line L587 (1.469, 2.112) -> (1.4692, 2.0978)
  line L588 (1.4692, 2.0978) -> (1.4689, 2.0837)
  line L589 (1.4689, 2.0837) -> (1.468, 2.0698)
  line L590 (1.468, 2.0698) -> (1.4672, 2.0629)
  line L591 (1.4672, 2.0629) -> (1.4668, 2.0595)
  line L592 (1.4668, 2.0595) -> (1.4663, 2.0561)
  line L593 (1.4663, 2.0561) -> (1.5188, 2.0344)
  line L594 (1.5188, 2.0344) -> (1.5208, 2.0371)
  line L595 (1.5208, 2.0371) -> (1.5229, 2.0398)
  line L596 (1.5229, 2.0398) -> (1.5273, 2.0452)
  line L597 (1.5273, 2.0452) -> (1.5364, 2.0557)
  line L598 (1.5364, 2.0557) -> (1.5461, 2.0659)
  line L599 (1.5461, 2.0659) -> (1.5564, 2.0759)
  line L600 (1.5564, 2.0759) -> (1.5671, 2.0856)
  line L601 (1.5671, 2.0856) -> (1.5783, 2.095)
  line L602 (1.5783, 2.095) -> (1.6252, 2.0711)
  line L603 (1.6252, 2.0711) -> (1.6241, 2.0565)
  line L604 (1.6241, 2.0565) -> (1.6226, 2.0421)
  line L605 (1.6226, 2.0421) -> (1.6205, 2.028)
  line L606 (1.6205, 2.028) -> (1.618, 2.0141)
  line L607 (1.618, 2.0141) -> (1.6149, 2.0006)
  line L608 (1.6149, 2.0006) -> (1.6131, 1.9939)
  line L609 (1.6131, 1.9939) -> (1.6121, 1.9906)
  line L610 (1.6121, 1.9906) -> (1.6112, 1.9873)
  line L611 (1.6112, 1.9873) -> (1.6595, 1.9577)
  line L612 (1.6595, 1.9577) -> (1.662, 1.9601)
  line L613 (1.662, 1.9601) -> (1.6645, 1.9624)
  line L614 (1.6645, 1.9624) -> (1.6696, 1.967)
  line L615 (1.6696, 1.967) -> (1.6803, 1.976)
  line L616 (1.6803, 1.976) -> (1.6915, 1.9845)
  line L617 (1.6915, 1.9845) -> (1.7032, 1.9927)
  line L618 (1.7032, 1.9927) -> (1.7153, 2.0006)
  line L619 (1.7153, 2.0006) -> (1.7278, 2.0082)
  line L620 (1.7278, 2.0082) -> (1.7704, 1.9773)
  line L621 (1.7704, 1.9773) -> (1.767, 1.963)
  line L622 (1.767, 1.963) -> (1.7633, 1.9491)
  line L623 (1.7633, 1.9491) -> (1.7591, 1.9354)
  line L624 (1.7591, 1.9354) -> (1.7544, 1.9221)
  line L625 (1.7544, 1.9221) -> (1.7492, 1.9092)
  line L626 (1.7492, 1.9092) -> (1.7464, 1.9029)
  line L627 (1.7464, 1.9029) -> (1.7449, 1.8998)
  line L628 (1.7449, 1.8998) -> (1.7434, 1.8967)
  line L629 (1.7434, 1.8967) -> (1.7866, 1.8599)
  line L630 (1.7866, 1.8599) -> (1.7894, 1.8619)
  line L631 (1.7894, 1.8619) -> (1.7922, 1.8638)
  line L632 (1.7922, 1.8638) -> (1.798, 1.8675)
  line L633 (1.798, 1.8675) -> (1.8099, 1.8747)
  line L634 (1.8099, 1.8747) -> (1.8223, 1.8814)
  line L635 (1.8223, 1.8814) -> (1.8352, 1.8877)
  line L636 (1.8352, 1.8877) -> (1.8484, 1.8936)
  line L637 (1.8484, 1.8936) -> (1.8619, 1.8991)
  line L638 (1.8619, 1.8991) -> (1.8991, 1.8619)
  line L639 (1.8991, 1.8619) -> (1.8936, 1.8484)
  line L640 (1.8936, 1.8484) -> (1.8877, 1.8352)
  line L641 (1.8877, 1.8352) -> (1.8814, 1.8223)
  line L642 (1.8814, 1.8223) -> (1.8747, 1.8099)
  line L643 (1.8747, 1.8099) -> (1.8675, 1.798)
  line L644 (1.8675, 1.798) -> (1.8638, 1.7922)
  line L645 (1.8638, 1.7922) -> (1.8619, 1.7894)
  line L646 (1.8619, 1.7894) -> (1.8599, 1.7866)
  line L647 (1.8599, 1.7866) -> (1.8967, 1.7434)
  line L648 (1.8967, 1.7434) -> (1.8998, 1.7449)
  line L649 (1.8998, 1.7449) -> (1.9029, 1.7464)
  line L650 (1.9029, 1.7464) -> (1.9092, 1.7492)
  line L651 (1.9092, 1.7492) -> (1.9221, 1.7544)
  line L652 (1.9221, 1.7544) -> (1.9354, 1.7591)
  line L653 (1.9354, 1.7591) -> (1.9491, 1.7633)
  line L654 (1.9491, 1.7633) -> (1.963, 1.767)
  line L655 (1.963, 1.767) -> (1.9773, 1.7704)
  line L656 (1.9773, 1.7704) -> (2.0082, 1.7278)
  line L657 (2.0082, 1.7278) -> (2.0006, 1.7153)
  line L658 (2.0006, 1.7153) -> (1.9927, 1.7032)
  line L659 (1.9927, 1.7032) -> (1.9845, 1.6915)
  line L660 (1.9845, 1.6915) -> (1.976, 1.6803)
  line L661 (1.976, 1.6803) -> (1.967, 1.6696)
  line L662 (1.967, 1.6696) -> (1.9624, 1.6645)
  line L663 (1.9624, 1.6645) -> (1.9601, 1.662)
  line L664 (1.9601, 1.662) -> (1.9577, 1.6595)
  line L665 (1.9577, 1.6595) -> (1.9873, 1.6112)
  line L666 (1.9873, 1.6112) -> (1.9906, 1.6121)
  line L667 (1.9906, 1.6121) -> (1.9939, 1.6131)
  line L668 (1.9939, 1.6131) -> (2.0006, 1.6149)
  line L669 (2.0006, 1.6149) -> (2.0141, 1.618)
  line L670 (2.0141, 1.618) -> (2.028, 1.6205)
  line L671 (2.028, 1.6205) -> (2.0421, 1.6226)
  line L672 (2.0421, 1.6226) -> (2.0565, 1.6241)
  line L673 (2.0565, 1.6241) -> (2.0711, 1.6252)
  line L674 (2.0711, 1.6252) -> (2.095, 1.5783)
  line L675 (2.095, 1.5783) -> (2.0856, 1.5671)
  line L676 (2.0856, 1.5671) -> (2.0759, 1.5564)
  line L677 (2.0759, 1.5564) -> (2.0659, 1.5461)
  line L678 (2.0659, 1.5461) -> (2.0557, 1.5364)
  line L679 (2.0557, 1.5364) -> (2.0452, 1.5273)
  line L680 (2.0452, 1.5273) -> (2.0398, 1.5229)
  line L681 (2.0398, 1.5229) -> (2.0371, 1.5208)
  line L682 (2.0371, 1.5208) -> (2.0344, 1.5188)
  line L683 (2.0344, 1.5188) -> (2.0561, 1.4663)
  line L684 (2.0561, 1.4663) -> (2.0595, 1.4668)
  line L685 (2.0595, 1.4668) -> (2.0629, 1.4672)
  line L686 (2.0629, 1.4672) -> (2.0698, 1.468)
  line L687 (2.0698, 1.468) -> (2.0837, 1.4689)
  line L688 (2.0837, 1.4689) -> (2.0978, 1.4692)
  line L689 (2.0978, 1.4692) -> (2.112, 1.469)
  line L690 (2.112, 1.469) -> (2.1265, 1.4683)
  line L691 (2.1265, 1.4683) -> (2.1411, 1.4671)
  line L692 (2.1411, 1.4671) -> (2.1573, 1.417)
  line L693 (2.1573, 1.417) -> (2.1462, 1.4075)
  line L694 (2.1462, 1.4075) -> (2.135, 1.3984)
  line L695 (2.135, 1.3984) -> (2.1236, 1.3898)
  line L696 (2.1236, 1.3898) -> (2.112, 1.3818)
  line L697 (2.112, 1.3818) -> (2.1002, 1.3744)
  line L698 (2.1002, 1.3744) -> (2.0942, 1.371)
  line L699 (2.0942, 1.371) -> (2.0912, 1.3693)
  line L700 (2.0912, 1.3693) -> (2.0882, 1.3677)
  line L701 (2.0882, 1.3677) -> (2.1014, 1.3125)
  line L702 (2.1014, 1.3125) -> (2.1048, 1.3125)
  line L703 (2.1048, 1.3125) -> (2.1083, 1.3124)
  line L704 (2.1083, 1.3124) -> (2.1151, 1.312)
  line L705 (2.1151, 1.312) -> (2.129, 1.3108)
  line L706 (2.129, 1.3108) -> (2.143, 1.3089)
  line L707 (2.143, 1.3089) -> (2.1571, 1.3065)
  line L708 (2.1571, 1.3065) -> (2.1712, 1.3035)
  line L709 (2.1712, 1.3035) -> (2.1854, 1.3)
  line L710 (2.1854, 1.3) -> (2.1936, 1.248)
  line L711 (2.1936, 1.248) -> (2.1812, 1.2403)
  line L712 (2.1812, 1.2403) -> (2.1687, 1.2331)
  line L713 (2.1687, 1.2331) -> (2.1561, 1.2264)
  line L714 (2.1561, 1.2264) -> (2.1433, 1.2203)
  line L715 (2.1433, 1.2203) -> (2.1305, 1.2149)
  line L716 (2.1305, 1.2149) -> (2.1241, 1.2124)
  line L717 (2.1241, 1.2124) -> (2.1209, 1.2112)
  line L718 (2.1209, 1.2112) -> (2.1176, 1.2101)
  line L719 (2.1176, 1.2101) -> (2.1221, 1.1536)
  line L720 (1.2517, 1.1017) -> (1.2466, 1.1405)
  line L721 (1.2466, 1.1405) -> (1.2316, 1.1767)
  line L722 (1.2316, 1.1767) -> (1.2078, 1.2078)
  line L723 (1.2078, 1.2078) -> (1.1767, 1.2316)
  line L724 (1.1767, 1.2316) -> (1.1405, 1.2466)
  line L725 (1.1405, 1.2466) -> (1.1017, 1.2517)
  line L726 (1.1017, 1.2517) -> (1.0629, 1.2466)
  line L727 (1.0629, 1.2466) -> (1.0267, 1.2316)
  line L728 (1.0267, 1.2316) -> (0.9956, 1.2078)
  line L729 (0.9956, 1.2078) -> (0.9718, 1.1767)
  line L730 (0.9718, 1.1767) -> (0.9568, 1.1405)
  line L731 (0.9568, 1.1405) -> (0.9517, 1.1017)
  line L732 (0.9517, 1.1017) -> (0.9568, 1.0629)
  line L733 (0.9568, 1.0629) -> (0.9718, 1.0267)
  line L734 (0.9718, 1.0267) -> (0.9956, 0.9956)
  line L735 (0.9956, 0.9956) -> (1.0267, 0.9718)
  line L736 (1.0267, 0.9718) -> (1.0629, 0.9568)
  line L737 (1.0629, 0.9568) -> (1.1017, 0.9517)
  line L738 (1.1017, 0.9517) -> (1.1405, 0.9568)
  line L739 (1.1405, 0.9568) -> (1.1767, 0.9718)
  line L740 (1.1767, 0.9718) -> (1.2078, 0.9956)
  line L741 (1.2078, 0.9956) -> (1.2316, 1.0267)
  line L742 (1.2316, 1.0267) -> (1.2466, 1.0629)
  line L743 (1.2466, 1.0629) -> (1.2517, 1.1017)
  point P0 (0, 0)
  constraints: 1488 end point
extrude "Extrusion1" add sketch "Sketch1" along normal blind 1